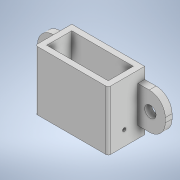
# Autodesk Inventor part: caixa do fusivel
Saved by Autodesk Inventor 2022 (Build 260153000, 153)
## iProperties
Created: 2022-03-30
Part Number: caixa do fusivel
Material: Genérico
Document SubType Name: Modeling
Designer: Hanter
Density: 1 g/cm^3
Appearance: Padrão
Author: Hanter
Autodesk Inventor part; units mm, degrees
ref_plane "YZ Plane" through (0, 0, 0) normal (1, 0, 0) x (0, 1, 0)
ref_plane "XZ Plane" through (0, 0, 0) normal (0, 1, 0) x (-1, 0, 0)
ref_plane "XY Plane" through (0, 0, 0) normal (0, 0, 1) x (1, 0, 0)
sketch "Esboço1" plane through (0, 0, 0) normal (0, 0, 1) x (1, 0, 0)
  line L0 (0, 0) -> (32, 0)
  line L1 (32, 0) -> (32, 26)
  line L2 (32, 26) -> (0, 26)
  line L3 (0, 26) -> (0, 0)
  dimension "d0" = 32
  dimension "d1" = 26
  constraints: 8 end point, 2 parallel, 1 horizontal, 1 perpendicular
  measures "d0" distance of L2.end L1.end
  measures "d1" distance of L1.end L0.end
extrude "Extrusão1" add sketch "Esboço1" against normal blind 16
shell "Casca1" thickness 2.5 removed faces 1 at (21.3333, 26, -10.6667)
sketch "Esboço2" plane through (0, 0, -16) normal (0, 0, -1) x (-1, 0, 0)
  line L0 (0, 0) -> (0, 26) projected
  line L1 (0, 21) -> (12, 21)
  line L2 (12, 21) -> (12, 5)
  line L3 (12, 5) -> (0, 5)
  line L4 (0, 5) -> (0, 21)
  line L5 (-32, 0) -> (0, 0) projected
  line L6 (-32, 26) -> (-32, 0) projected
  line L7 (-32, 21) -> (-44, 21)
  line L8 (-44, 21) -> (-44, 5)
  line L9 (-44, 5) -> (-32, 5)
  line L10 (-32, 5) -> (-32, 21)
  point P0 (-32, 5)
  point P1 (0, 5)
  dimension "d5" = 12
  dimension "d6" = 16
  dimension "d7" = 5
  dimension "d8" = 12
  dimension "d18" = 16
  dimension "d19" = 5
  constraints: 16 end point, 4 parallel, 2 horizontal, 2 perpendicular, 2 point on line
  measures "d5" distance of L2.end L3.end
  measures "d6" distance of L1.end L2.end
  measures "d7" distance between parallel lines of L5 L3
  measures "d8" distance of L9.end L8.end
  measures "d18" distance of L7.end L8.end
  measures "d19" distance between parallel lines of L5 L9
extrude "Extrusão2" add sketch "Esboço2" against normal blind 3
sketch "Esboço3" plane through (0, 0, -16) normal (0, 0, -1) x (-1, 0, 0)
  circle A0 centre (5.5, 13) radius 2.5
  line L0 (12, 5) -> (12, 21) projected
  circle A1 centre (-37.5, 13) radius 2.5
  line L1 (-44, 21) -> (-44, 5) projected
  point P0 (0, 0)
  dimension "d11" = 5
  dimension "d12" = 6.5
  dimension "d13" = 5
  dimension "d14" = 6.5
  constraints: 2 centre point
  measures "d11" diameter of A0
  measures "d12" distance from line of L0 A0.centre
  measures "d13" diameter of A1
  measures "d14" distance from line of L1 A1.centre
extrude "Extrusão3" cut sketch "Esboço3" against normal blind 3
fillet "Arredondamento1" radius 7 4 edges at (44, 21, -14.5) (44, 5, -14.5) (-12, 5, -14.5) (-12, 21, -14.5)
fillet "Arredondamento2" radius 1 2 edges at (32, 13, 0) (0, 13, 0)
sketch "Esboço4" plane through (32, 5, -13) normal (1, 0, 0) x (0, 0, -1)
  circle A0 centre (-6, 1.428) radius 0.75
  line L0 (0, 0) -> (0, 7) projected
  point P0 (-13, -5)
  dimension "d21" = 1.5
  dimension "d22" = 6
  constraints: 1 centre point
  measures "d21" diameter of A0
  measures "d22" distance from line of L0 A0.centre
extrude "Extrusão4" cut sketch "Esboço4" against normal blind 36.75
